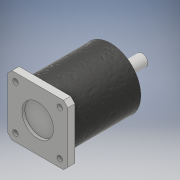
# Autodesk Inventor part: 911-42-reducer-long
Saved by Autodesk Inventor 2018 (Build 220112000, 112)
## iProperties
Created: 2019-12-10
Part Number: 911-42-reducer-long
Material: Generic
Document SubType Name: Modeling
Designer: Bunny320
Density: 1 g/cm^3
Appearance: Default
Author: Bunny320
Autodesk Inventor part; units mm, degrees
ref_plane "YZ Plane" through (0, 0, 0) normal (1, 0, 0) x (0, 1, 0)
ref_plane "XZ Plane" through (0, 0, 0) normal (0, 1, 0) x (-1, 0, 0)
ref_plane "XY Plane" through (0, 0, 0) normal (0, 0, 1) x (1, 0, 0)
sketch "Sketch1" plane through (0, 0, 0) normal (0, 1, 0) x (-1, 0, 0)
  line L0 (-21, -21) -> (21, -21)
  line L1 (21, -21) -> (21, 21)
  line L2 (21, 21) -> (-21, 21)
  line L3 (-21, 21) -> (-21, -21)
  line L4 (-21, -21) -> (21, 21) construction
  line L5 (21, -21) -> (-21, 21) construction
  point P0 (0, 0)
  dimension "d0" = 42
  constraints: 12 end point, 2 midpoint, 2 parallel, 2 perpendicular, 1 horizontal
  measures "d0" distance of L1.end L2.end
extrude "Extrusion1" add sketch "Sketch1" along normal blind 5
sketch "Sketch2" plane through (0, 0, 0) normal (0, 1, 0) x (1, 0, 0)
  circle A0 centre (0, 0) radius 21
  dimension "d3" = 42
  constraints: 1 centre point, 1 coincident
  measures "d3" diameter of A0
extrude "Extrusion2" add sketch "Sketch2" along normal blind 51
sketch "Sketch3" plane through (0, 51, 0) normal (0, 1, 0) x (1, 0, 0)
  circle A0 centre (0, 0) radius 12.5
  dimension "d6" = 25
  constraints: 1 centre point, 1 coincident
  measures "d6" diameter of A0
extrude "Extrusion3" add sketch "Sketch3" along normal blind 2
sketch "Sketch4" plane through (0, 51, 0) normal (0, 1, 0) x (1, 0, 0)
  circle A0 centre (0, 0) radius 4
  dimension "d9" = 8
  constraints: 1 centre point, 1 coincident
  measures "d9" diameter of A0
extrude "Extrusion4" add sketch "Sketch4" along normal blind 22
sketch "Sketch5" plane through (0, 51, 0) normal (0, 1, 0) x (1, 0, 0)
  line L0 (-12.3744, -12.3744) -> (12.3744, -12.3744)
  line L1 (12.3744, -12.3744) -> (12.3744, 12.3744)
  line L2 (12.3744, 12.3744) -> (-12.3744, 12.3744)
  line L3 (-12.3744, 12.3744) -> (-12.3744, -12.3744)
  line L4 (-12.3744, -12.3744) -> (12.3744, 12.3744) construction
  line L5 (12.3744, -12.3744) -> (-12.3744, 12.3744) construction
  point P0 (0, 0)
  dimension "d15" = 35
  constraints: 12 end point, 4 coincident, 2 midpoint, 2 parallel, 2 perpendicular, 1 horizontal
  measures "d15" distance of L0.end L2.end
hole "Hole1" at (12.3744, 51, -12.3744) at (-12.3744, 51, -12.3744) at (-12.3744, 51, 12.3744) at (12.3744, 51, 12.3744) direction (0, -1, 0) diameter 3.242 depth 6 tip angle 118 thread size "M4x0.7" class "6H" standard "ISO Metric profile"
sketch "Sketch6" plane through (0, 73, 0) normal (0, 1, 0) x (1, 0, 0)
  point P0 (0, 0)
  point P1 (0, 0)
  constraints: 1 coincident
hole "Hole2" at (0, 73, 0) direction (0, -1, 0) diameter 2.459 depth 6 tip angle 118 thread size "M3x0.5" class "6H" standard "ISO Metric profile"
chamfer "Chamfer1" distance 3 angle 45 4 edges at (21, 2.5, -21) (-21, 2.5, -21) (21, 2.5, 21) (-21, 2.5, 21)
sketch "Sketch7" plane through (0, 0, 0) normal (0, 1, 0) x (-1, 0, 0)
  circle A0 centre (0, 0) radius 11
  dimension "d30" = 22
  constraints: 1 centre point, 1 coincident
  measures "d30" diameter of A0
extrude "Extrusion5" cut sketch "Sketch7" along normal blind 2
sketch "Sketch8" plane through (0, 0, 0) normal (0, 1, 0) x (-1, 0, 0)
  line L0 (15.5, 15.5) -> (-15.5, 15.5)
  line L1 (-15.5, 15.5) -> (-15.5, -15.5)
  line L2 (-15.5, -15.5) -> (15.5, -15.5)
  line L3 (15.5, -15.5) -> (15.5, 15.5)
  line L4 (15.5, 15.5) -> (-15.5, -15.5) construction
  line L5 (-15.5, 15.5) -> (15.5, -15.5) construction
  point P0 (0, 0)
  dimension "d33" = 31
  constraints: 12 end point, 4 coincident, 2 midpoint, 2 parallel, 2 perpendicular, 1 horizontal
  measures "d33" distance of L0.end L1.end
hole "Hole3" at (15.5, 0, 15.5) at (-15.5, 0, 15.5) at (-15.5, 0, -15.5) at (15.5, 0, -15.5) direction (0, 1, 0) diameter 3.7 depth 5
sketch "Sketch9" plane through (0, 5, 0) normal (0, 1, 0) x (1, 0, 0)
  arc A0 (-15.9176, -13.6978) -> (-13.6978, -15.9176) centre (-15.5, -15.5) ccw projected
  circle A1 centre (-15.5, 15.5) radius 1.85 projected
  arc A2 (15.9176, 13.6978) -> (13.6978, 15.9176) centre (15.5, 15.5) ccw projected
  circle A3 centre (15.5, -15.5) radius 1.85 projected
  point P0 (0, 0)
  constraints: 4 coincident
body "Solid1"
